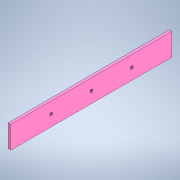
# Autodesk Inventor part: Pestaña
Saved by Autodesk Inventor 2022.6 (Build 266554000, 554)
## iProperties
Created: 2025-01-16
Part Number: Pestaña
Material: Genérico
Document SubType Name: Modeling
Designer: johan
Density: 1 g/cm^3
Appearance: Valor por defecto
Author: johan
Autodesk Inventor part; units mm, degrees
ref_plane "YZ Plane" through (0, 0, 0) normal (1, 0, 0) x (0, 1, 0)
ref_plane "XZ Plane" through (0, 0, 0) normal (0, 1, 0) x (-1, 0, 0)
ref_plane "XY Plane" through (0, 0, 0) normal (0, 0, 1) x (1, 0, 0)
sketch "Boceto1" plane through (0, 0, 0) normal (1, 0, 0) x (0, 1, 0)
  line L0 (0, 0) -> (25, 0)
  line L1 (25, 0) -> (25, -180)
  line L2 (25, -180) -> (0, -180)
  line L3 (0, -180) -> (0, 0)
  dimension "d0" = 25
  dimension "d1" = 180
  constraints: 8 end point, 2 parallel, 1 horizontal, 1 perpendicular
  measures "d0" distance of L1.end L2.end
  measures "d1" distance of L0.end L1.end
extrude "Extrusión1" add sketch "Boceto1" along normal blind 3
sketch "Boceto2" plane through (3, 0, 0) normal (1, 0, 0) x (0, 0, -1)
  line L0 (180, 0) -> (180, 25) projected
  line L1 (180, 25) -> (0, 25) projected
  line L2 (0, 25) -> (0, 0) projected
  line L3 (0, 0) -> (180, 0) projected
  circle A0 centre (45, 12.5) radius 1.5875
  circle A1 centre (90, 12.5) radius 1.5875
  circle A2 centre (135, 12.5) radius 1.5875
  dimension "d4" = 3.175
  dimension "d5" = 45
  dimension "d8" = 45
  dimension "d15" = 45
  constraints: 3 centre point, 2 horizontal, 4 other
  measures "d4" diameter of A0
  measures "d5" distance from line of L2 A0.centre
  measures "d8" distance of A0.centre A1.centre
  measures "d15" distance of A1.centre A2.centre
extrude "Extrusión2" cut sketch "Boceto2" against normal blind 3 contours A0 | A1 | A2
